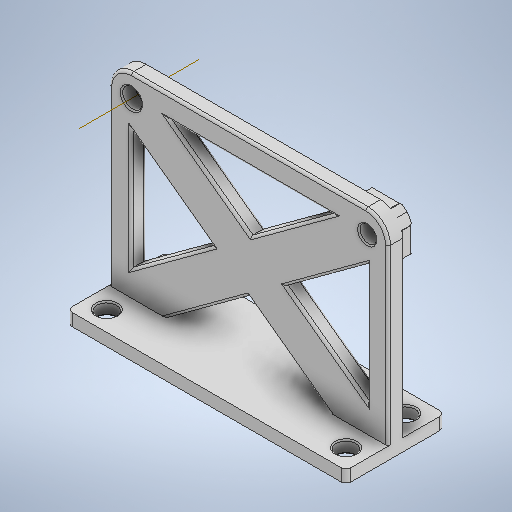
# Autodesk Inventor part: Steering Mounting Plate
Saved by Autodesk Inventor 2025.2 (Build 292293000, 293)
## iProperties
Created: 2025-02-04
Part Number: Steering Mounting Plate
Material: Generic
Document SubType Name: Modeling
Designer: eason
Density: 1 g/cm^3
Appearance: Default
Author: eason
Autodesk Inventor part; units mm, degrees
ref_plane "YZ Plane" through (0, 0, 0) normal (1, 0, 0) x (0, 1, 0)
ref_plane "XZ Plane" through (0, 0, 0) normal (0, 1, 0) x (-1, 0, 0)
ref_plane "XY Plane" through (0, 0, 0) normal (0, 0, 1) x (1, 0, 0)
sketch "Sketch1" plane through (0, 0, 0) normal (0, 0, 1) x (1, 0, 0)
  circle A0 centre (0, 0) radius 4
  circle A1 centre (95.5, 0) radius 3.4
  line L0 (-34.1895, 0) -> (129.0895, 0) projected
  line L1 (0, 9) -> (94.9, 9)
  line L2 (103.9, 0) -> (103.9, -75)
  line L3 (103.9, -75) -> (-9, -75)
  line L4 (-9, -75) -> (-9, 0)
  line L5 (0, 4) -> (-4, 4) construction
  line L6 (-4, 4) -> (-4, 0) construction
  line L7 (95.5, 3.4) -> (98.9, 3.4) construction
  line L8 (98.9, 3.4) -> (98.9, 0) construction
  arc A2 (0, 9) -> (-9, 0) centre (0, 0) ccw
  arc A3 (103.9, 0) -> (94.9, 9) centre (94.9, 0) ccw
  line L9 (-9, -75) -> (103.9, -75)
  line L10 (103.9, -75) -> (103.9, -70)
  line L11 (103.9, -70) -> (-9, -70)
  line L12 (-9, -70) -> (-9, -75)
  arc A4 (87.1, 0) -> (95.5, -8.4) centre (95.5, 0) ccw
  line L13 (9, 0) -> (87.1, 0)
  line L14 (95.5, -8.4) -> (95.5, -70)
  line L15 (0, -9) -> (0, -70)
  arc A5 (0, -9) -> (9, 0) centre (0, 0) ccw
  arc A6 (0, 9) -> (-9, 0) centre (0, 0) ccw
  line L16 (0, 0) -> (95.5, -70) construction
  line L17 (95.5, 0) -> (0, -70) construction
  line L18 (15.2238, 0) -> (95.5, -58.8412)
  line L19 (80.2762, -70) -> (0, -11.1588)
  line L20 (81.2911, 0) -> (0, -59.5851)
  line L21 (95.5, -10.4149) -> (14.2089, -70)
  point P0 (-9, -70)
  point P1 (47.2425, -45.7868)
  point P2 (48.2575, -24.2132)
  point P3 (33.0337, -35.372)
  point P4 (62.4663, -34.628)
  dimension "d0" = 95.5
  dimension "d1" = 6.8
  dimension "d2" = 8
  dimension "d3" = 75
  dimension "d4" = 5
  dimension "d5" = 5
  dimension "d6" = 5
  dimension "d7" = 5
  dimension "d8" = 8.4
  dimension "d9" = 9
  constraints: 42 end point, 14 point on circle, 12 point on line, 12 tangent, 8 parallel, 7 centre point, 4 horizontal, 4 perpendicular, 3 coincident, 9 other
  measures "d0" distance of point (0, 0) A1.centre
  measures "d1" diameter of A1
  measures "d2" diameter of A0
  measures "d3" distance from line of L3 point (0, 0)
  measures "d4" distance between parallel lines of L5 L1
  measures "d5" distance between parallel lines of L4 L6
  measures "d6" distance between parallel lines of L2 L8
  measures "d7" distance between parallel lines of L3 L11
  measures "d8" radius of A4
  measures "d9" radius of A5
extrude "Extrusion1" add sketch "Sketch1" along normal mid plane 6 contours L0 A5 L15 L11 L4 A0 | A0 L0 A2 L1 A3 A1 | L0 L18 L20 L19 L15 A5 | L0 A4 L14 L21 L18 L20 | L18 L21 L19 L20 | L15 L20 L19 L21 L11 | L0 A1 L2 L11 L14 A4 | L18 L14 L11 L19 L21
extrude "Extrusion2" add sketch "Sketch1" along normal mid plane 40 contours L11 L2 L3 L4
sketch "Sketch2" plane through (-9, -75, 20) normal (0, -1, 0) x (1, 0, 0)
  circle A0 centre (104.9, -32) radius 4
  circle A1 centre (104.9, -8) radius 4
  circle A2 centre (8, -32) radius 4
  circle A3 centre (8, -8) radius 4
  line L0 (112.9, -40) -> (0, -40) projected
  line L1 (112.9, -40) -> (112.9, 0) projected
  line L2 (0, 0) -> (112.9, 0) projected
  line L3 (0, -40) -> (0, 0) projected
  point P0 (9, -20)
  dimension "d14" = 8
  dimension "d15" = 8
  dimension "d16" = 8
  dimension "d17" = 8
  dimension "d18" = 8
  dimension "d19" = 8
  dimension "d20" = 8
  dimension "d21" = 8
  dimension "d22" = 8
  dimension "d23" = 8
  dimension "d24" = 8
  dimension "d25" = 8
  constraints: 4 centre point
  measures "d14" diameter of A0
  measures "d15" diameter of A1
  measures "d16" diameter of A2
  measures "d17" diameter of A3
  measures "d18" distance from line of L0 A0.centre
  measures "d19" distance from line of L1 A0.centre
  measures "d20" distance from line of L2 A1.centre
  measures "d21" distance from line of L1 A1.centre
  measures "d22" distance from line of L3 A3.centre
  measures "d23" distance from line of L2 A3.centre
  measures "d24" distance from line of L0 A2.centre
  measures "d25" distance from line of L3 A2.centre
extrude "Extrusion3" cut sketch "Sketch2" against normal up to surface (5 mm away) contours A0 | A1 | A2 | A3
fillet "Fillet1" radius 2 4 edges at (103.9, -72.5, -20) (-9, -72.5, -20) (-9, -72.5, 20) (103.9, -72.5, 20)
fillet "Fillet2" radius 1 27 edges at (101.264, 6.364, 3) (47.45, 9, 3) (-6.364, 6.364, 3) (-9, -35, 3) (103.9, -35, 3) (64.7743, -12.1066, -3) (64.7743, -12.1066, 3) (48.2575, 0, -3) (31.7406, -12.1066, 3) (31.7406, -12.1066, -3) (48.2575, 0, 3) (16.5168, -23.2654, -3) (16.5168, -23.2654, 3) (16.5168, -47.4785, -3) (16.5168, -47.4785, 3) (0, -35.372, -3) (0, -35.372, 3) (78.9832, -22.5215, -3) (78.9832, -22.5215, 3) (78.9832, -46.7346, -3) (78.9832, -46.7346, 3) (95.5, -34.628, 3) (95.5, -34.628, -3) (63.7594, -57.8934, -3) (63.7594, -57.8934, 3) (30.7257, -57.8934, -3) (30.7257, -57.8934, 3)
fillet "Fillet3" radius 0.5 12 edges at (92.1, 0, -3) (92.1, 0, 3) (-4, 0, 3) (-4, 0, -3) (-5, -70, 12) (-5, -75, 12) (91.9, -70, 12) (91.9, -75, 12) (91.9, -70, -12) (91.9, -75, -12) (-5, -70, -12) (-5, -75, -12)
sketch "Sketch3" plane through (0, 0, -3) normal (0, 0, -1) x (-1, 0, 0)
  line L0 (-101.55, 6) -> (-89.45, 6)
  line L1 (-89.45, 6) -> (-89.45, -6)
  line L2 (-89.45, -6) -> (-101.55, -6)
  line L3 (-101.55, -6) -> (-101.55, 6)
  line L4 (-101.55, 6) -> (-89.45, -6) construction
  line L5 (-89.45, 6) -> (-101.55, -6) construction
  circle A0 centre (-95.5, 0) radius 4.3882
  circle A1 centre (-95.5, 0) radius 3.9 projected
  line L6 (-87.45, 8) -> (-87.45, -8)
  line L7 (-87.45, -8) -> (-103.55, -8)
  line L8 (-103.55, 7.9835) -> (-103.55, 8)
  line L9 (-103.55, -8) -> (-103.55, 2.5302)
  line L10 (-87.45, 8) -> (-99.0231, 8)
  arc A2 (-94.9, 9) -> (-103.9, 0) centre (-94.9, 0) ccw projected
  point P0 (0, 0)
  point P1 (-103.55, 2.4855)
  dimension "d31" = 12
  dimension "d32" = 12.1
  dimension "d35" = 2
  dimension "d36" = 2
  dimension "d37" = 2
  dimension "d38" = 2
  constraints: 22 end point, 5 parallel, 1 centre point, 1 coincident, 1 concentric, 1 horizontal, 1 midpoint, 1 perpendicular, 1 point on circle, 1 point on line
  measures "d31" distance between parallel lines of L2 L0
  measures "d32" distance between parallel lines of L3 L1
  measures "d35" distance between parallel lines of L1 L6
  measures "d36" distance between parallel lines of L2 L7
  measures "d37" distance between parallel lines of L9 L3
  measures "d38" distance between parallel lines of L0 L10
extrude "Extrusion4" add sketch "Sketch3" along normal blind 4 contours L6 L7 L9 A2 L10
fillet "Fillet4" radius 0.2 4 edges at (101.55, 0, -7) (95.5, 6, -7) (89.45, 0, -7) (95.5, -6, -7)
fillet "Fillet5" radius 0.5 9 edges at (103.55, -8, -5) (87.45, -8, -5) (87.45, 8, -5) (99.0231, 8, -5) (103.55, 2.4855, -5) (87.45, 0, -7) (93.2366, 8, -7) (103.55, -2.7573, -7) (95.5, -8, -7)
body "Solid1"
